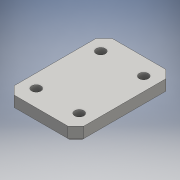
# Autodesk Inventor part: camera_adapter
Saved by Autodesk Inventor 2016 (Build 200138000, 138)
## iProperties
Created: 2016-02-09
Part Number: camera_adapter
Material: Generic
Document SubType Name: Modeling
Designer: element
Density: 1 g/cm^3
Appearance: Default
Mass: 4.25107 g
Surface Area: 25.9904 cm^2
Volume: 4.25107 cm^3
Author: element
Autodesk Inventor part; units mm, degrees
ref_plane "YZ Plane" through (0, 0, 0) normal (1, 0, 0) x (0, 1, 0)
ref_plane "XZ Plane" through (0, 0, 0) normal (0, 1, 0) x (-1, 0, 0)
ref_plane "XY Plane" through (0, 0, 0) normal (0, 0, 1) x (1, 0, 0)
sketch "Sketch1" plane through (0, 0, 0) normal (0, 0, 1) x (1, 0, 0)
  line L0 (0, 0) -> (-26, 0)
  line L1 (0, 0) -> (0, 36.5)
  line L2 (0, 36.5) -> (-26, 36.5)
  line L3 (-26, 36.5) -> (-26, 0)
  dimension "d0" = 26
  dimension "d1" = 36.5
  constraints: 8 end point, 2 horizontal, 1 perpendicular, 1 vertical
  measures "d0" distance of L0.start L0.end
  measures "d1" distance of L0.start L1.end
sketch "Sketch2" plane through (0, 0, 0) normal (0, 0, 1) x (1, 0, 0)
  line L0 (-13, 0) -> (-13, 6.25)
  circle A0 centre (-21, 30.25) radius 1.7
  circle A1 centre (-21, 6.25) radius 1.7
  circle A2 centre (-5, 30.25) radius 1.7
  circle A3 centre (-5, 6.25) radius 1.7
  line L1 (-13, 6.25) -> (-5, 6.25)
  line L2 (-13, 6.25) -> (-21, 6.25)
  line L3 (-21, 30.25) -> (-5, 30.25)
  line L4 (-5, 30.25) -> (-5, 6.25)
  line L5 (-21, 18.25) -> (-13, 18.25)
  line L6 (-13, 18.25) -> (-13, 6.25)
  line L7 (-21, 6.25) -> (-21, 18.25)
  line L8 (-21, 18.25) -> (-21, 30.25)
  line L9 (0, 0) -> (-13, 0)
  line L10 (-18.075, 4.5613) -> (-21, 2.8725)
  line L11 (-21, 2.8725) -> (-23.925, 4.5613)
  line L12 (-23.925, 4.5613) -> (-23.925, 7.9387)
  line L13 (-23.925, 7.9387) -> (-21, 9.6275)
  line L14 (-21, 9.6275) -> (-18.075, 7.9387)
  line L15 (-18.075, 7.9387) -> (-18.075, 4.5613)
  line L16 (-7.925, 7.9387) -> (-5, 9.6275)
  line L17 (-5, 9.6275) -> (-2.075, 7.9387)
  line L18 (-2.075, 7.9387) -> (-2.075, 4.5613)
  line L19 (-2.075, 4.5613) -> (-5, 2.8725)
  line L20 (-5, 2.8725) -> (-7.925, 4.5613)
  line L21 (-7.925, 4.5613) -> (-7.925, 7.9387)
  line L22 (-7.925, 31.9387) -> (-5, 33.6275)
  line L23 (-5, 33.6275) -> (-2.075, 31.9387)
  line L24 (-2.075, 31.9387) -> (-2.075, 28.5613)
  line L25 (-2.075, 28.5613) -> (-5, 26.8725)
  line L26 (-5, 26.8725) -> (-7.925, 28.5613)
  line L27 (-7.925, 28.5613) -> (-7.925, 31.9387)
  line L28 (-18.075, 28.5613) -> (-21, 26.8725)
  line L29 (-21, 26.8725) -> (-23.925, 28.5613)
  line L30 (-23.925, 28.5613) -> (-23.925, 31.9387)
  line L31 (-23.925, 31.9387) -> (-21, 33.6275)
  line L32 (-21, 33.6275) -> (-18.075, 31.9387)
  line L33 (-18.075, 31.9387) -> (-18.075, 28.5613)
  point P0 (8.2274, 51.4671)
  point P1 (-18.075, 6.25)
  point P2 (-7.925, 6.25)
  point P3 (-7.925, 30.25)
  point P4 (-18.075, 30.25)
  dimension "d2" = 3.4
  dimension "d3" = 3.4
  dimension "d4" = 3.4
  dimension "d5" = 3.4
  dimension "d7" = 8
  dimension "d8" = 8
  dimension "d9" = 12
  dimension "d10" = 12
  dimension "d12" = 18.25
  dimension "d13" = 13
  dimension "d34" = 5.85
  dimension "d35" = 5.85
  dimension "d36" = 5.85
  dimension "d37" = 5.85
  constraints: 68 end point, 12 coincident, 5 point on line, 4 centre point, 4 horizontal, 4 midpoint, 2 perpendicular, 2 vertical, 1 collinear, 52 other
  measures "d2" diameter of A0
  measures "d3" diameter of A2
  measures "d4" diameter of A3
  measures "d5" diameter of A1
  measures "d7" distance of L0.end L2.end
  measures "d8" distance of L0.end L1.end
  measures "d9" distance between parallel lines of L2 L5
  measures "d10" distance of L5.start L3.start
  measures "d12" distance of L0.start L5.end
  measures "d13" distance of L9.start L0.start
  measures "d34" distance between parallel lines of L15 L12
  measures "d35" distance between parallel lines of L18 L21
  measures "d36" distance between parallel lines of L24 L27
  measures "d37" distance between parallel lines of L33 L30
extrude "Extrusion1" add sketch "Sketch1" along normal blind 5
hole "Hole1" at (8.2274, 51.4671, 0) at (-5, 30.25, 0) at (-21, 30.25, 0) at (-21, 6.25, 0) at (-5, 6.25, 0) direction (0, 0, 1) diameter 3.4 end through all
chamfer "Chamfer1" distance 3 angle 45 4 edges at (0, 0, 2.5) (-26, 0, 2.5) (-26, 36.5, 2.5) (0, 36.5, 2.5)
extrude "Extrusion3" cut sketch "Sketch2" along normal blind 2 contours L3 L33 L28 L8 A0 | A0 L8 L29 L30 L31 L32 L33 L3 | L27 L22 L23 L24 L25 L4 A2 L3 | L3 A2 L4 L26 L27 | L14 L15 L2 A1 L7 | L7 A1 L2 L15 L10 L11 L12 L13 | L17 L18 L19 L20 L21 L1 A3 L4 | L4 A3 L1 L21 L16
chamfer "Chamfer2" distance 1 angle 45 8 edges at (-1.5, 1.5, 0) (-13, 0, 0) (-24.5, 1.5, 0) (-26, 18.25, 0) (-13, 36.5, 0) (-1.5, 35, 0) (-24.5, 35, 0) (0, 18.25, 0)
equation "\"d3\" = d2"
equation "\"d4\" = d2"
equation "\"d5\" = d2"
equation "\"d8\" = d7"
equation "\"d9\" = d10"
equation "\"d13\" = 0.5 * d0"
equation "\"d35\" = d34"
equation "\"d36\" = d34"
equation "\"d37\" = d34"
equation "\"d16\" = d2"
body "Solid1"
